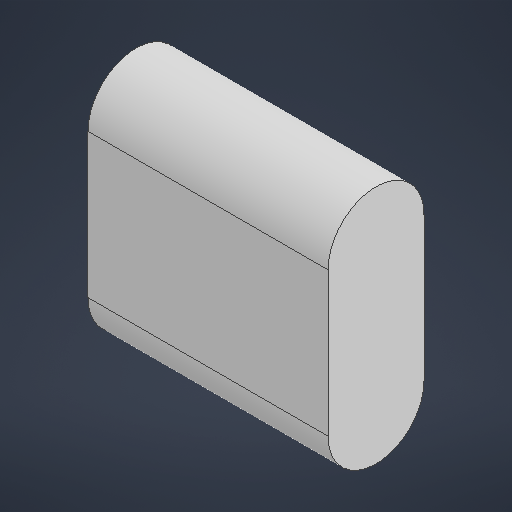
# Autodesk Inventor part: Lock Tab
Saved by Autodesk Inventor 2026.1 (Build 301233000, 233)
## iProperties
Created: 2026-06-29
Part Number: Lock Tab
Material: Generic
Document SubType Name: Modeling
Designer: share
Density: 1 g/cm^3
Appearance: Default
Author: share
Autodesk Inventor part; units mm, degrees
ref_plane "YZ Plane" through (0, 0, 0) normal (1, 0, 0) x (0, 1, 0)
ref_plane "XZ Plane" through (0, 0, 0) normal (0, 1, 0) x (-1, 0, 0)
ref_plane "XY Plane" through (0, 0, 0) normal (0, 0, 1) x (1, 0, 0)
sketch "Sketch1" plane through (0, 0, 0) normal (1, 0, 0) x (0, 1, 0)
  arc A0 (3.6208, -2) -> (3.6208, 2) centre (3.6208, 0) ccw
  arc A1 (-2.3792, 2) -> (-2.3792, -2) centre (-2.3792, 0) ccw
  line L0 (0, 2.8) -> (0, -2.8) construction
  line L1 (-6.3792, 0) -> (7.6208, 0) construction
  line L2 (3.6208, 0) -> (-2.3792, 0) construction
  line L3 (3.6208, 2) -> (-2.3792, 2)
  line L4 (-2.3792, -2) -> (3.6208, -2)
  point P0 (0, 0)
  dimension "d0" = 2
  dimension "d1" = 6
  constraints: 6 end point, 4 point on circle, 2 centre point, 2 collinear, 2 tangent, 1 equal radius, 1 horizontal
  measures "d0" radius of A0
  measures "d1" distance of L2.end L2.start
extrude "Extrusion1" add sketch "Sketch1" along normal blind 10
body "Solid1"
